Autodesk Fusion 360 part; units mm, degrees
note: some values were not read from the file. Set by a fixed rule: which sketch regions a step uses.
(part 2 of 2)
sketch "Sketch31" plane through (0, 0, 44.392) normal (0, 0, 1) x (-1, 0, 0)
  line L0 (5, 0) -> (10, 0)
  line L1 (10, 0) -> (10, 5)
  line L2 (10, 5) -> (5, 5)
  line L3 (5, 5) -> (5, 0)
  line L4 (5, 5) -> (6.35, 5)
  line L5 (6.35, 5) -> (6.35, 3.65)
  line L6 (6.35, 3.65) -> (5, 3.65)
  line L7 (5, 3.65) -> (5, 5)
  line L8 (6.35, 3.65) -> (8.65, 3.65)
  line L9 (8.65, 3.65) -> (8.65, 1.35)
  line L10 (8.65, 1.35) -> (6.35, 1.35)
  line L11 (6.35, 1.35) -> (6.35, 3.65)
  line L12 (5, -65) -> (6.35, -65)
  line L13 (6.35, -65) -> (6.35, -63.65)
  line L14 (6.35, -63.65) -> (5, -63.65)
  line L15 (5, -63.65) -> (5, -65)
  line L16 (6.35, -63.65) -> (8.65, -63.65)
  line L17 (8.65, -63.65) -> (8.65, -61.35)
  line L18 (8.65, -61.35) -> (6.35, -61.35)
  line L19 (6.35, -61.35) -> (6.35, -63.65)
  dimension "d193" = 1.35
  dimension "d194" = 1.35
  dimension "d195" = 2.3
  dimension "d196" = 2.3
  dimension "d197" = 1.35
  dimension "d198" = 1.35
  dimension "d199" = 2.3
  dimension "d200" = 2.3
  constraint horizontal L4
  constraint vertical L5
  constraint horizontal L6
  constraint vertical L7
  constraint coincident L2.end L3.start
  constraint horizontal L8
  constraint vertical L9
  constraint horizontal L10
  constraint vertical L11
  constraint horizontal L12
  constraint vertical L13
  constraint horizontal L14
  constraint vertical L15
  constraint horizontal L16
  constraint vertical L17
  constraint horizontal L18
  constraint vertical L19
  measures "d193" distance of L2.end L4.end
  measures "d194" distance of L2.end L6.end
  measures "d195" distance of L5.end L8.end
  measures "d196" distance of L5.end L10.end
  measures "d197" distance of L12.start L12.end
  measures "d198" distance of L12.start L14.end
  measures "d199" distance of L13.end L16.end
  measures "d200" distance of L13.end L18.end
extrude "Extrude29" add sketch "Sketch31" along normal blind 5 contours L8 L9 L10 L11 | L16 L17 L18 L19
sketch "Sketch32" plane through (0, -5, 0) normal (0, -1, 0) x (1, 0, 0)
